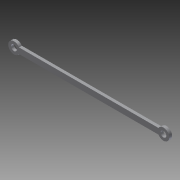
# Autodesk Inventor part: bar2
Saved by Autodesk Inventor 2011 (Build 150239000, 239)
## iProperties
Created: 2011-07-10
Part Number: bar2
Document SubType Name: Modeling
Designer: adowning
Density: 1 g/cm^3
Author: adowning
Autodesk Inventor part; units mm, degrees
ref_plane "YZ Plane" through (0, 0, 0) normal (1, 0, 0) x (0, 1, 0)
ref_plane "XZ Plane" through (0, 0, 0) normal (0, 1, 0) x (-1, 0, 0)
ref_plane "XY Plane" through (0, 0, 0) normal (0, 0, 1) x (1, 0, 0)
sketch "Sketch1" plane through (0, 0, 0) normal (0, 0, 1) x (1, 0, 0)
  line L0 (-42.1338, 2.3056) -> (122.9662, 2.3056)
  line L1 (122.9662, 2.3056) -> (122.9662, -4.0444)
  line L2 (122.9662, -4.0444) -> (-42.1338, -4.0444)
  line L3 (-42.1338, -4.0444) -> (-42.1338, 2.3056)
  line L4 (-42.1338, 2.3056) -> (-42.1338, -0.8694)
  line L5 (-42.1338, -0.8694) -> (122.9662, -0.8694)
  circle A0 centre (-42.1338, -0.8694) radius 3.175
  circle A1 centre (122.9662, -0.8694) radius 3.175
  point P0 (0, 0)
  dimension "d0" = 165.1
  dimension "d1" = 6.35
  constraints: 12 end point, 2 coincident, 2 midpoint, 2 parallel, 1 centre point, 1 horizontal, 1 perpendicular, 1 tangent, 1 vertical alignment, 2 other
  measures "d0" distance of L1.end L2.end
  measures "d1" distance of L0.end L1.end
extrude "Extrusion1" add sketch "Sketch1" along normal blind 3.175
sketch "Sketch2" plane through (0, 0, 3.175) normal (0, 0, 1) x (1, 0, 0)
  arc A0 (122.9662, -4.0444) -> (122.9662, 2.3056) centre (122.9662, -0.8694) ccw projected
  arc A1 (-42.1338, 2.3056) -> (-42.1338, -4.0444) centre (-42.1338, -0.8694) ccw projected
  circle A2 centre (-42.1338, -0.8694) radius 3.175
  circle A3 centre (122.9662, -0.8694) radius 6.35
  circle A4 centre (-42.1338, -0.8694) radius 6.35
  circle A5 centre (122.9662, -0.8694) radius 3.175
  point P0 (0, 0)
  dimension "d4" = 12.7
  dimension "d5" = 12.7
  constraints: 4 coincident, 2 centre point, 2 vertical alignment, 4 other
  measures "d4" diameter of A3
  measures "d5" diameter of A4
extrude "Extrusion2" cut sketch "Sketch2" against normal blind 3.175 contours A5 A0 | A2 A1
sketch "Sketch3" plane through (0, 0, 3.175) normal (0, 0, 1) x (1, 0, 0)
  arc A0 (122.9662, 2.3056) -> (122.9662, -4.0444) centre (122.9662, -0.8694) ccw projected
  arc A1 (-42.1338, -4.0444) -> (-42.1338, 2.3056) centre (-42.1338, -0.8694) ccw projected
  circle A2 centre (-42.1338, -0.8694) radius 3.175
  circle A3 centre (-42.1338, -0.8694) radius 6.35
  circle A4 centre (122.9662, -0.8694) radius 3.175
  circle A5 centre (122.9662, -0.8694) radius 6.35
  point P0 (0, 0)
  dimension "d8" = 12.7
  dimension "d9" = 12.7
  constraints: 4 coincident, 2 centre point, 2 vertical alignment, 4 other
  measures "d8" diameter of A3
  measures "d9" diameter of A5
extrude "Extrusion3" add sketch "Sketch3" against normal blind 3.175
body "Solid1"
